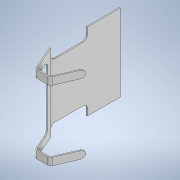
# Autodesk Inventor part: armor_top
Saved by Autodesk Inventor 2021 (Build 250183000, 183)
## iProperties
Created: 2022-05-15
Part Number: armor_top
Material: Generic
Document SubType Name: Modeling
Designer: ermoz
Density: 1 g/cm^3
Appearance: Default
Author: ermoz
Autodesk Inventor part; units mm, degrees
ref_plane "YZ Plane" through (0, 0, 0) normal (1, 0, 0) x (0, 1, 0)
ref_plane "XZ Plane" through (0, 0, 0) normal (0, 1, 0) x (-1, 0, 0)
sketch "Sketch1" plane through (0, 0, 0) normal (0, 1, 0) x (-1, 0, 0)
  line L0 (0, 0) -> (1.5, 0)
  line L1 (1.5, 0) -> (1.5, 95)
  line L2 (1.5, 95) -> (0, 95)
  line L3 (0, 95) -> (0, 0)
  line L4 (1.5, 95) -> (-13.6286, 130)
  line L5 (-13.6286, 130) -> (-33.6286, 130)
  line L6 (-33.6286, 130) -> (-48.5, 95.5952)
  line L7 (-48.5, 95.5952) -> (-47.1231, 95)
  line L8 (-47.1231, 95) -> (-32.6429, 128.5)
  line L9 (-32.6429, 128.5) -> (-14.4803, 128.5)
  line L10 (-14.4803, 128.5) -> (0, 95)
  dimension "d0" = 1.5
  dimension "d1" = 95
  dimension "d3" = 1.5
  dimension "d4" = 1.5
  dimension "d5" = 20
  dimension "d6" = 50
  dimension "d21" = 35
  constraints: 22 end point, 5 parallel, 2 horizontal, 2 perpendicular, 1 equal length, 1 horizontal alignment
  measures "d0" distance of L0.start L0.end
  measures "d1" distance of L0.end L1.end
  measures "d3" distance between parallel lines of L5 L9
  measures "d4" distance between parallel lines of L8 L6
  measures "d5" distance of L4.end L5.end
  measures "d6" distance from line of L6.end L1
  measures "d21" distance between parallel lines of L2 L5
extrude "Extrusion1" add sketch "Sketch1" along normal blind 105
ref_plane "Work Plane1" through (0, 95, 0) normal (0, 1, 0) x (1, 0, 0)
sketch "Sketch2" plane through (0, 95, 0) normal (0, 1, 0) x (1, 0, 0)
  line L0 (0, -95) -> (54.3942, -95)
  line L1 (54.3942, -95) -> (54.3942, -147.6515)
  line L2 (54.3942, -147.6515) -> (3.3148, -147.6515)
  line L3 (-1.5, 0) -> (-1.5, -95) projected
  line L4 (-0.9211, -95.4972) -> (3.3148, -95.4972)
  line L5 (3.3148, -95.4972) -> (3.3148, -147.6515)
  line L6 (14.4803, -128.5) -> (0, -95) projected
  line L7 (3.3148, -102.6689) -> (1.8148, -102.6689)
  line L8 (-1.5, -95) -> (13.6286, -130) projected
  line L9 (1.8148, -102.6689) -> (1.8148, -137.9948)
  line L10 (1.8148, -137.9948) -> (3.3148, -137.9948)
  point P0 (3.3886, -95)
  point P1 (13.6286, -130)
  point P2 (0.2149, -95.4972)
  constraints: 16 end point, 3 horizontal, 3 point on line, 2 perpendicular, 2 vertical, 1 parallel, 2 other
extrude "Extrusion2" cut sketch "Sketch2" against normal blind 85 contours L0 L1 L2 L5 L4 L6 | L5 L8 L7 | L5 L10 L9 L8
fillet "Fillet1" radius 2.5 4 edges at (14.4803, 100, 128.5) (32.6429, 100, 128.5) (32.6429, 5, 128.5) (14.4803, 5, 128.5)
fillet "Fillet2" radius 4 5 edges at (-1.5, 52.5, 95) (13.6286, 100, 130) (33.6286, 100, 130) (33.6286, 5, 130) (13.6286, 5, 130)
sketch "Sketch3" plane through (-1.5, 0, 0) normal (-1, 0, 0) x (0, 0, 1)
  line L0 (45, 0) -> (95, 0)
  line L1 (95, 0) -> (95, 15)
  line L2 (95, 15) -> (45, 15)
  line L3 (45, 15) -> (45, 0)
  line L4 (45, 90) -> (95, 90)
  line L5 (95, 90) -> (95, 105)
  line L6 (95, 105) -> (45, 105)
  line L7 (45, 105) -> (45, 90)
  line L8 (0, 105) -> (94.1725, 105) projected
  line L9 (0, 0) -> (94.1725, 0) projected
  line L10 (0, 0) -> (0, 105) projected
  dimension "d15" = 50
  dimension "d16" = 15
  dimension "d17" = 45
  constraints: 16 end point, 4 parallel, 3 collinear, 2 horizontal, 2 perpendicular, 2 point on line
  measures "d15" distance of L0.start L0.end
  measures "d16" distance of L2.end L0.start
  measures "d17" distance between parallel lines of L10 L3
extrude "Extrusion3" cut sketch "Sketch3" against normal blind 65
fillet "Fillet3" radius 6 10 edges at (2.5648, 10, 102.6689) (2.5648, 95, 102.6689) (-0.75, 90, 45) (-0.7067, 90, 95) (-0.7067, 15, 95) (-0.75, 15, 45) (47.8116, 105, 95.2976) (47.8116, 95, 95.2976) (47.8116, 0, 95.2976) (47.8116, 10, 95.2976)
body "Solid1"
